Autodesk Inventor part; units mm, degrees
(part 4 of 15)
  line L606 (16.684, 10.808) -> (18.716, 10.808)
  arc A1487 (18.716, 10.7572) -> (18.716, 10.8588) centre (18.716, 10.808) ccw
  arc A1488 (16.684, 10.8588) -> (16.684, 10.7572) centre (16.684, 10.808) ccw
  line L607 (18.716, 10.808) -> (18.716, 9.792)
  arc A1489 (18.6652, 9.792) -> (18.7668, 9.792) centre (18.716, 9.792) ccw
  arc A1490 (18.7668, 10.808) -> (18.6652, 10.808) centre (18.716, 10.808) ccw
  line L608 (18.716, 9.792) -> (16.684, 9.792)
  arc A1491 (16.684, 9.8428) -> (16.684, 9.7412) centre (16.684, 9.792) ccw
  arc A1492 (18.716, 9.7412) -> (18.716, 9.8428) centre (18.716, 9.792) ccw
  line L609 (16.684, 9.792) -> (16.684, 10.808)
  arc A1493 (16.7348, 10.808) -> (16.6332, 10.808) centre (16.684, 10.808) ccw
  arc A1494 (16.6332, 9.792) -> (16.7348, 9.792) centre (16.684, 9.792) ccw
  arc A1495 (39.1348, 45.008) -> (39.0332, 45.008) centre (39.084, 45.008) ccw
  line L610 (22.884, 6.808) -> (24.916, 6.808)
  arc A1496 (24.916, 6.7572) -> (24.916, 6.8588) centre (24.916, 6.808) ccw
  arc A1497 (22.884, 6.8588) -> (22.884, 6.7572) centre (22.884, 6.808) ccw
  line L611 (24.916, 6.808) -> (24.916, 5.792)
  arc A1498 (24.8652, 5.792) -> (24.9668, 5.792) centre (24.916, 5.792) ccw
  arc A1499 (24.9668, 6.808) -> (24.8652, 6.808) centre (24.916, 6.808) ccw
  line L612 (24.916, 5.792) -> (22.884, 5.792)
  arc A1500 (22.884, 5.8428) -> (22.884, 5.7412) centre (22.884, 5.792) ccw
  arc A1501 (24.916, 5.7412) -> (24.916, 5.8428) centre (24.916, 5.792) ccw
  line L613 (22.884, 5.792) -> (22.884, 6.808)
  arc A1502 (22.9348, 6.808) -> (22.8332, 6.808) centre (22.884, 6.808) ccw
  arc A1503 (22.8332, 5.792) -> (22.9348, 5.792) centre (22.884, 5.792) ccw
  arc A1504 (39.0332, 43.992) -> (39.1348, 43.992) centre (39.084, 43.992) ccw
  line L614 (12.684, 13.208) -> (14.716, 13.208)
  arc A1505 (14.716, 13.1572) -> (14.716, 13.2588) centre (14.716, 13.208) ccw
  arc A1506 (12.684, 13.2588) -> (12.684, 13.1572) centre (12.684, 13.208) ccw
  line L615 (14.716, 13.208) -> (14.716, 12.192)
  arc A1507 (14.6652, 12.192) -> (14.7668, 12.192) centre (14.716, 12.192) ccw
  arc A1508 (14.7668, 13.208) -> (14.6652, 13.208) centre (14.716, 13.208) ccw
  line L616 (14.716, 12.192) -> (12.684, 12.192)
  arc A1509 (12.684, 12.2428) -> (12.684, 12.1412) centre (12.684, 12.192) ccw
  arc A1510 (14.716, 12.1412) -> (14.716, 12.2428) centre (14.716, 12.192) ccw
  line L617 (12.684, 12.192) -> (12.684, 13.208)
  arc A1511 (12.7348, 13.208) -> (12.6332, 13.208) centre (12.684, 13.208) ccw
  arc A1512 (12.6332, 12.192) -> (12.7348, 12.192) centre (12.684, 12.192) ccw
  line L618 (39.084, 45.008) -> (41.116, 45.008)
  line L619 (14.684, 13.208) -> (16.716, 13.208)
  arc A1513 (16.716, 13.1572) -> (16.716, 13.2588) centre (16.716, 13.208) ccw
  arc A1514 (14.684, 13.2588) -> (14.684, 13.1572) centre (14.684, 13.208) ccw
  line L620 (16.716, 13.208) -> (16.716, 12.192)
  arc A1515 (16.6652, 12.192) -> (16.7668, 12.192) centre (16.716, 12.192) ccw
  arc A1516 (16.7668, 13.208) -> (16.6652, 13.208) centre (16.716, 13.208) ccw
  line L621 (16.716, 12.192) -> (14.684, 12.192)
  arc A1517 (14.684, 12.2428) -> (14.684, 12.1412) centre (14.684, 12.192) ccw
  arc A1518 (16.716, 12.1412) -> (16.716, 12.2428) centre (16.716, 12.192) ccw
  line L622 (14.684, 12.192) -> (14.684, 13.208)
  arc A1519 (14.7348, 13.208) -> (14.6332, 13.208) centre (14.684, 13.208) ccw
  arc A1520 (14.6332, 12.192) -> (14.7348, 12.192) centre (14.684, 12.192) ccw
  arc A1521 (41.116, 44.9572) -> (41.116, 45.0588) centre (41.116, 45.008) ccw
  line L623 (12.684, 21.208) -> (14.716, 21.208)
  arc A1522 (14.716, 21.1572) -> (14.716, 21.2588) centre (14.716, 21.208) ccw
  arc A1523 (12.684, 21.2588) -> (12.684, 21.1572) centre (12.684, 21.208) ccw
  line L624 (14.716, 21.208) -> (14.716, 20.192)
  arc A1524 (14.6652, 20.192) -> (14.7668, 20.192) centre (14.716, 20.192) ccw
  arc A1525 (14.7668, 21.208) -> (14.6652, 21.208) centre (14.716, 21.208) ccw
  line L625 (14.716, 20.192) -> (12.684, 20.192)
  arc A1526 (12.684, 20.2428) -> (12.684, 20.1412) centre (12.684, 20.192) ccw
  arc A1527 (14.716, 20.1412) -> (14.716, 20.2428) centre (14.716, 20.192) ccw
  line L626 (12.684, 20.192) -> (12.684, 21.208)
  arc A1528 (12.7348, 21.208) -> (12.6332, 21.208) centre (12.684, 21.208) ccw
  arc A1529 (12.6332, 20.192) -> (12.7348, 20.192) centre (12.684, 20.192) ccw
  arc A1530 (39.084, 45.0588) -> (39.084, 44.9572) centre (39.084, 45.008) ccw
  line L627 (12.684, 2.808) -> (14.716, 2.808)
  arc A1531 (14.716, 2.7572) -> (14.716, 2.8588) centre (14.716, 2.808) ccw
  arc A1532 (12.684, 2.8588) -> (12.684, 2.7572) centre (12.684, 2.808) ccw
  line L628 (14.716, 2.808) -> (14.716, 1.792)
  arc A1533 (14.6652, 1.792) -> (14.7668, 1.792) centre (14.716, 1.792) ccw
  arc A1534 (14.7668, 2.808) -> (14.6652, 2.808) centre (14.716, 2.808) ccw
  line L629 (14.716, 1.792) -> (12.684, 1.792)
  arc A1535 (12.684, 1.8428) -> (12.684, 1.7412) centre (12.684, 1.792) ccw
  arc A1536 (14.716, 1.7412) -> (14.716, 1.8428) centre (14.716, 1.792) ccw
  line L630 (12.684, 1.792) -> (12.684, 2.808)
  arc A1537 (12.7348, 2.808) -> (12.6332, 2.808) centre (12.684, 2.808) ccw
  arc A1538 (12.6332, 1.792) -> (12.7348, 1.792) centre (12.684, 1.792) ccw
  line L631 (41.116, 45.008) -> (41.116, 43.992)
  line L632 (14.684, 2.808) -> (16.716, 2.808)
  arc A1539 (16.716, 2.7572) -> (16.716, 2.8588) centre (16.716, 2.808) ccw
  arc A1540 (14.684, 2.8588) -> (14.684, 2.7572) centre (14.684, 2.808) ccw
  line L633 (16.716, 2.808) -> (16.716, 1.792)
  arc A1541 (16.6652, 1.792) -> (16.7668, 1.792) centre (16.716, 1.792) ccw
  arc A1542 (16.7668, 2.808) -> (16.6652, 2.808) centre (16.716, 2.808) ccw
  line L634 (16.716, 1.792) -> (14.684, 1.792)
  arc A1543 (14.684, 1.8428) -> (14.684, 1.7412) centre (14.684, 1.792) ccw
  arc A1544 (16.716, 1.7412) -> (16.716, 1.8428) centre (16.716, 1.792) ccw
  line L635 (14.684, 1.792) -> (14.684, 2.808)
  arc A1545 (14.7348, 2.808) -> (14.6332, 2.808) centre (14.684, 2.808) ccw
  arc A1546 (14.6332, 1.792) -> (14.7348, 1.792) centre (14.684, 1.792) ccw
  arc A1547 (41.0652, 43.992) -> (41.1668, 43.992) centre (41.116, 43.992) ccw
  line L636 (12.684, 10.808) -> (14.716, 10.808)
  arc A1548 (14.716, 10.7572) -> (14.716, 10.8588) centre (14.716, 10.808) ccw
  arc A1549 (12.684, 10.8588) -> (12.684, 10.7572) centre (12.684, 10.808) ccw
  line L637 (14.716, 10.808) -> (14.716, 9.792)
  arc A1550 (14.6652, 9.792) -> (14.7668, 9.792) centre (14.716, 9.792) ccw
  arc A1551 (14.7668, 10.808) -> (14.6652, 10.808) centre (14.716, 10.808) ccw
  line L638 (14.716, 9.792) -> (12.684, 9.792)
  arc A1552 (12.684, 9.8428) -> (12.684, 9.7412) centre (12.684, 9.792) ccw
  arc A1553 (14.716, 9.7412) -> (14.716, 9.8428) centre (14.716, 9.792) ccw
  line L639 (12.684, 9.792) -> (12.684, 10.808)
  arc A1554 (12.7348, 10.808) -> (12.6332, 10.808) centre (12.684, 10.808) ccw
  arc A1555 (12.6332, 9.792) -> (12.7348, 9.792) centre (12.684, 9.792) ccw
  arc A1556 (41.1668, 45.008) -> (41.0652, 45.008) centre (41.116, 45.008) ccw
  line L640 (14.684, 21.208) -> (16.716, 21.208)
  arc A1557 (16.716, 21.1572) -> (16.716, 21.2588) centre (16.716, 21.208) ccw
  arc A1558 (14.684, 21.2588) -> (14.684, 21.1572) centre (14.684, 21.208) ccw
  line L641 (16.716, 21.208) -> (16.716, 20.192)
  arc A1559 (16.6652, 20.192) -> (16.7668, 20.192) centre (16.716, 20.192) ccw
  arc A1560 (16.7668, 21.208) -> (16.6652, 21.208) centre (16.716, 21.208) ccw
  line L642 (16.716, 20.192) -> (14.684, 20.192)
  arc A1561 (14.684, 20.2428) -> (14.684, 20.1412) centre (14.684, 20.192) ccw
  arc A1562 (16.716, 20.1412) -> (16.716, 20.2428) centre (16.716, 20.192) ccw
  line L643 (14.684, 20.192) -> (14.684, 21.208)
  arc A1563 (14.7348, 21.208) -> (14.6332, 21.208) centre (14.684, 21.208) ccw
  arc A1564 (14.6332, 20.192) -> (14.7348, 20.192) centre (14.684, 20.192) ccw
  line L644 (41.116, 42.992) -> (39.084, 42.992)
  line L645 (16.716, 16.192) -> (14.684, 16.192)
  arc A1565 (14.684, 16.2428) -> (14.684, 16.1412) centre (14.684, 16.192) ccw
  arc A1566 (16.716, 16.1412) -> (16.716, 16.2428) centre (16.716, 16.192) ccw
  line L646 (14.684, 16.192) -> (14.684, 17.208)
  arc A1567 (14.7348, 17.208) -> (14.6332, 17.208) centre (14.684, 17.208) ccw
  arc A1568 (14.6332, 16.192) -> (14.7348, 16.192) centre (14.684, 16.192) ccw
  line L647 (14.684, 17.208) -> (16.716, 17.208)
  arc A1569 (16.716, 17.1572) -> (16.716, 17.2588) centre (16.716, 17.208) ccw
  arc A1570 (14.684, 17.2588) -> (14.684, 17.1572) centre (14.684, 17.208) ccw
  line L648 (16.716, 17.208) -> (16.716, 16.192)
  arc A1571 (16.6652, 16.192) -> (16.7668, 16.192) centre (16.716, 16.192) ccw
  arc A1572 (16.7668, 17.208) -> (16.6652, 17.208) centre (16.716, 17.208) ccw
  arc A1573 (39.084, 43.0428) -> (39.084, 42.9412) centre (39.084, 42.992) ccw
  line L649 (22.884, 13.208) -> (24.916, 13.208)
  arc A1574 (24.916, 13.1572) -> (24.916, 13.2588) centre (24.916, 13.208) ccw
  arc A1575 (22.884, 13.2588) -> (22.884, 13.1572) centre (22.884, 13.208) ccw
  line L650 (24.916, 13.208) -> (24.916, 12.192)
  arc A1576 (24.8652, 12.192) -> (24.9668, 12.192) centre (24.916, 12.192) ccw
  arc A1577 (24.9668, 13.208) -> (24.8652, 13.208) centre (24.916, 13.208) ccw
  line L651 (24.916, 12.192) -> (22.884, 12.192)
  arc A1578 (22.884, 12.2428) -> (22.884, 12.1412) centre (22.884, 12.192) ccw
  arc A1579 (24.916, 12.1412) -> (24.916, 12.2428) centre (24.916, 12.192) ccw
  line L652 (22.884, 12.192) -> (22.884, 13.208)
  arc A1580 (22.9348, 13.208) -> (22.8332, 13.208) centre (22.884, 13.208) ccw
  arc A1581 (22.8332, 12.192) -> (22.9348, 12.192) centre (22.884, 12.192) ccw
  arc A1582 (41.116, 42.9412) -> (41.116, 43.0428) centre (41.116, 42.992) ccw
  line L653 (14.684, 10.808) -> (16.716, 10.808)
  arc A1583 (16.716, 10.7572) -> (16.716, 10.8588) centre (16.716, 10.808) ccw
  arc A1584 (14.684, 10.8588) -> (14.684, 10.7572) centre (14.684, 10.808) ccw
  line L654 (16.716, 10.808) -> (16.716, 9.792)
  arc A1585 (16.6652, 9.792) -> (16.7668, 9.792) centre (16.716, 9.792) ccw
  arc A1586 (16.7668, 10.808) -> (16.6652, 10.808) centre (16.716, 10.808) ccw
  line L655 (16.716, 9.792) -> (14.684, 9.792)
  arc A1587 (14.684, 9.8428) -> (14.684, 9.7412) centre (14.684, 9.792) ccw
  arc A1588 (16.716, 9.7412) -> (16.716, 9.8428) centre (16.716, 9.792) ccw
  line L656 (14.684, 9.792) -> (14.684, 10.808)
  arc A1589 (14.7348, 10.808) -> (14.6332, 10.808) centre (14.684, 10.808) ccw
  arc A1590 (14.6332, 9.792) -> (14.7348, 9.792) centre (14.684, 9.792) ccw
  line L657 (39.084, 42.992) -> (39.084, 44.008)
  line L658 (16.716, 5.692) -> (14.684, 5.692)
  arc A1591 (14.684, 5.7428) -> (14.684, 5.6412) centre (14.684, 5.692) ccw
  arc A1592 (16.716, 5.6412) -> (16.716, 5.7428) centre (16.716, 5.692) ccw
  line L659 (14.684, 5.692) -> (14.684, 6.708)
  arc A1593 (14.7348, 6.708) -> (14.6332, 6.708) centre (14.684, 6.708) ccw
  arc A1594 (14.6332, 5.692) -> (14.7348, 5.692) centre (14.684, 5.692) ccw
  line L660 (14.684, 6.708) -> (16.716, 6.708)
  arc A1595 (16.716, 6.6572) -> (16.716, 6.7588) centre (16.716, 6.708) ccw
  arc A1596 (14.684, 6.7588) -> (14.684, 6.6572) centre (14.684, 6.708) ccw
  line L661 (16.716, 6.708) -> (16.716, 5.692)
  arc A1597 (16.6652, 5.692) -> (16.7668, 5.692) centre (16.716, 5.692) ccw
  arc A1598 (16.7668, 6.708) -> (16.6652, 6.708) centre (16.716, 6.708) ccw
  arc A1599 (39.1348, 44.008) -> (39.0332, 44.008) centre (39.084, 44.008) ccw
  line L662 (22.884, 2.808) -> (24.916, 2.808)
  arc A1600 (24.916, 2.7572) -> (24.916, 2.8588) centre (24.916, 2.808) ccw
  arc A1601 (22.884, 2.8588) -> (22.884, 2.7572) centre (22.884, 2.808) ccw
  line L663 (24.916, 2.808) -> (24.916, 1.792)
  arc A1602 (24.8652, 1.792) -> (24.9668, 1.792) centre (24.916, 1.792) ccw
  arc A1603 (24.9668, 2.808) -> (24.8652, 2.808) centre (24.916, 2.808) ccw
  line L664 (24.916, 1.792) -> (22.884, 1.792)
  arc A1604 (22.884, 1.8428) -> (22.884, 1.7412) centre (22.884, 1.792) ccw
  arc A1605 (24.916, 1.7412) -> (24.916, 1.8428) centre (24.916, 1.792) ccw
  line L665 (22.884, 1.792) -> (22.884, 2.808)
  arc A1606 (22.9348, 2.808) -> (22.8332, 2.808) centre (22.884, 2.808) ccw
  arc A1607 (22.8332, 1.792) -> (22.9348, 1.792) centre (22.884, 1.792) ccw
  arc A1608 (39.0332, 42.992) -> (39.1348, 42.992) centre (39.084, 42.992) ccw
  line L666 (20.916, 12.192) -> (18.884, 12.192)
  arc A1609 (18.884, 12.2428) -> (18.884, 12.1412) centre (18.884, 12.192) ccw
  arc A1610 (20.916, 12.1412) -> (20.916, 12.2428) centre (20.916, 12.192) ccw
  line L667 (18.884, 12.192) -> (18.884, 13.208)
  arc A1611 (18.9348, 13.208) -> (18.8332, 13.208) centre (18.884, 13.208) ccw
  arc A1612 (18.8332, 12.192) -> (18.9348, 12.192) centre (18.884, 12.192) ccw
  line L668 (18.884, 13.208) -> (20.916, 13.208)
  arc A1613 (20.916, 13.1572) -> (20.916, 13.2588) centre (20.916, 13.208) ccw
  arc A1614 (18.884, 13.2588) -> (18.884, 13.1572) centre (18.884, 13.208) ccw
  line L669 (20.916, 13.208) -> (20.916, 12.192)
  arc A1615 (20.8652, 12.192) -> (20.9668, 12.192) centre (20.916, 12.192) ccw
  arc A1616 (20.9668, 13.208) -> (20.8652, 13.208) centre (20.916, 13.208) ccw
  line L670 (39.084, 44.008) -> (41.116, 44.008)
  line L671 (12.684, 17.208) -> (14.716, 17.208)
  arc A1617 (14.716, 17.1572) -> (14.716, 17.2588) centre (14.716, 17.208) ccw
  arc A1618 (12.684, 17.2588) -> (12.684, 17.1572) centre (12.684, 17.208) ccw
  line L672 (14.716, 17.208) -> (14.716, 16.192)
  arc A1619 (14.6652, 16.192) -> (14.7668, 16.192) centre (14.716, 16.192) ccw
  arc A1620 (14.7668, 17.208) -> (14.6652, 17.208) centre (14.716, 17.208) ccw
  line L673 (14.716, 16.192) -> (12.684, 16.192)
  arc A1621 (12.684, 16.2428) -> (12.684, 16.1412) centre (12.684, 16.192) ccw
  arc A1622 (14.716, 16.1412) -> (14.716, 16.2428) centre (14.716, 16.192) ccw
  line L674 (12.684, 16.192) -> (12.684, 17.208)
  arc A1623 (12.7348, 17.208) -> (12.6332, 17.208) centre (12.684, 17.208) ccw
  arc A1624 (12.6332, 16.192) -> (12.7348, 16.192) centre (12.684, 16.192) ccw
  arc A1625 (41.116, 43.9572) -> (41.116, 44.0588) centre (41.116, 44.008) ccw
  line L675 (20.884, 21.208) -> (22.916, 21.208)
  arc A1626 (22.916, 21.1572) -> (22.916, 21.2588) centre (22.916, 21.208) ccw
  arc A1627 (20.884, 21.2588) -> (20.884, 21.1572) centre (20.884, 21.208) ccw
  line L676 (22.916, 21.208) -> (22.916, 20.192)
  arc A1628 (22.8652, 20.192) -> (22.9668, 20.192) centre (22.916, 20.192) ccw
  arc A1629 (22.9668, 21.208) -> (22.8652, 21.208) centre (22.916, 21.208) ccw
  line L677 (22.916, 20.192) -> (20.884, 20.192)
  arc A1630 (20.884, 20.2428) -> (20.884, 20.1412) centre (20.884, 20.192) ccw
  arc A1631 (22.916, 20.1412) -> (22.916, 20.2428) centre (22.916, 20.192) ccw
  line L678 (20.884, 20.192) -> (20.884, 21.208)
  arc A1632 (20.9348, 21.208) -> (20.8332, 21.208) centre (20.884, 21.208) ccw
  arc A1633 (20.8332, 20.192) -> (20.9348, 20.192) centre (20.884, 20.192) ccw
  arc A1634 (39.084, 44.0588) -> (39.084, 43.9572) centre (39.084, 44.008) ccw
  line L679 (18.884, 2.808) -> (20.916, 2.808)
  arc A1635 (20.916, 2.7572) -> (20.916, 2.8588) centre (20.916, 2.808) ccw
  arc A1636 (18.884, 2.8588) -> (18.884, 2.7572) centre (18.884, 2.808) ccw
  line L680 (20.916, 2.808) -> (20.916, 1.792)
  arc A1637 (20.8652, 1.792) -> (20.9668, 1.792) centre (20.916, 1.792) ccw
  arc A1638 (20.9668, 2.808) -> (20.8652, 2.808) centre (20.916, 2.808) ccw
  line L681 (20.916, 1.792) -> (18.884, 1.792)
  arc A1639 (18.884, 1.8428) -> (18.884, 1.7412) centre (18.884, 1.792) ccw
  arc A1640 (20.916, 1.7412) -> (20.916, 1.8428) centre (20.916, 1.792) ccw
  line L682 (18.884, 1.792) -> (18.884, 2.808)
  arc A1641 (18.9348, 2.808) -> (18.8332, 2.808) centre (18.884, 2.808) ccw
  arc A1642 (18.8332, 1.792) -> (18.9348, 1.792) centre (18.884, 1.792) ccw
  line L683 (41.116, 44.008) -> (41.116, 42.992)
  line L684 (12.684, 6.708) -> (14.716, 6.708)
  arc A1643 (14.716, 6.6572) -> (14.716, 6.7588) centre (14.716, 6.708) ccw
  arc A1644 (12.684, 6.7588) -> (12.684, 6.6572) centre (12.684, 6.708) ccw
  line L685 (14.716, 6.708) -> (14.716, 5.692)
  arc A1645 (14.6652, 5.692) -> (14.7668, 5.692) centre (14.716, 5.692) ccw
  arc A1646 (14.7668, 6.708) -> (14.6652, 6.708) centre (14.716, 6.708) ccw
  line L686 (14.716, 5.692) -> (12.684, 5.692)
  arc A1647 (12.684, 5.7428) -> (12.684, 5.6412) centre (12.684, 5.692) ccw
  arc A1648 (14.716, 5.6412) -> (14.716, 5.7428) centre (14.716, 5.692) ccw
  line L687 (12.684, 5.692) -> (12.684, 6.708)
  arc A1649 (12.7348, 6.708) -> (12.6332, 6.708) centre (12.684, 6.708) ccw
  arc A1650 (12.6332, 5.692) -> (12.7348, 5.692) centre (12.684, 5.692) ccw
  arc A1651 (41.0652, 42.992) -> (41.1668, 42.992) centre (41.116, 42.992) ccw
  line L688 (20.884, 10.808) -> (22.916, 10.808)
  arc A1652 (22.916, 10.7572) -> (22.916, 10.8588) centre (22.916, 10.808) ccw
  arc A1653 (20.884, 10.8588) -> (20.884, 10.7572) centre (20.884, 10.808) ccw
  line L689 (22.916, 10.808) -> (22.916, 9.792)
  arc A1654 (22.8652, 9.792) -> (22.9668, 9.792) centre (22.916, 9.792) ccw
  arc A1655 (22.9668, 10.808) -> (22.8652, 10.808) centre (22.916, 10.808) ccw
  line L690 (22.916, 9.792) -> (20.884, 9.792)
  arc A1656 (20.884, 9.8428) -> (20.884, 9.7412) centre (20.884, 9.792) ccw
  arc A1657 (22.916, 9.7412) -> (22.916, 9.8428) centre (22.916, 9.792) ccw
  line L691 (20.884, 9.792) -> (20.884, 10.808)
  arc A1658 (20.9348, 10.808) -> (20.8332, 10.808) centre (20.884, 10.808) ccw
  arc A1659 (20.8332, 9.792) -> (20.9348, 9.792) centre (20.884, 9.792) ccw
  arc A1660 (41.1668, 44.008) -> (41.0652, 44.008) centre (41.116, 44.008) ccw
  line L692 (22.884, 21.208) -> (24.916, 21.208)
  arc A1661 (24.916, 21.1572) -> (24.916, 21.2588) centre (24.916, 21.208) ccw
  arc A1662 (22.884, 21.2588) -> (22.884, 21.1572) centre (22.884, 21.208) ccw
  line L693 (24.916, 21.208) -> (24.916, 20.192)
  arc A1663 (24.8652, 20.192) -> (24.9668, 20.192) centre (24.916, 20.192) ccw
  arc A1664 (24.9668, 21.208) -> (24.8652, 21.208) centre (24.916, 21.208) ccw
  line L694 (24.916, 20.192) -> (22.884, 20.192)
  arc A1665 (22.884, 20.2428) -> (22.884, 20.1412) centre (22.884, 20.192) ccw
  arc A1666 (24.916, 20.1412) -> (24.916, 20.2428) centre (24.916, 20.192) ccw
  line L695 (22.884, 20.192) -> (22.884, 21.208)
  arc A1667 (22.9348, 21.208) -> (22.8332, 21.208) centre (22.884, 21.208) ccw
  arc A1668 (22.8332, 20.192) -> (22.9348, 20.192) centre (22.884, 20.192) ccw
  line L696 (68.816, 35.092) -> (66.784, 35.092)
  line L697 (18.684, 17.208) -> (20.716, 17.208)
  arc A1669 (20.716, 17.1572) -> (20.716, 17.2588) centre (20.716, 17.208) ccw
  arc A1670 (18.684, 17.2588) -> (18.684, 17.1572) centre (18.684, 17.208) ccw
  line L698 (20.716, 17.208) -> (20.716, 16.192)
  arc A1671 (20.6652, 16.192) -> (20.7668, 16.192) centre (20.716, 16.192) ccw
  arc A1672 (20.7668, 17.208) -> (20.6652, 17.208) centre (20.716, 17.208) ccw
  line L699 (20.716, 16.192) -> (18.684, 16.192)
  arc A1673 (18.684, 16.2428) -> (18.684, 16.1412) centre (18.684, 16.192) ccw
  arc A1674 (20.716, 16.1412) -> (20.716, 16.2428) centre (20.716, 16.192) ccw
  line L700 (18.684, 16.192) -> (18.684, 17.208)
  arc A1675 (18.7348, 17.208) -> (18.6332, 17.208) centre (18.684, 17.208) ccw
  arc A1676 (18.6332, 16.192) -> (18.7348, 16.192) centre (18.684, 16.192) ccw
  arc A1677 (66.784, 35.1428) -> (66.784, 35.0412) centre (66.784, 35.092) ccw
  line L701 (22.884, 10.808) -> (24.916, 10.808)
  arc A1678 (24.916, 10.7572) -> (24.916, 10.8588) centre (24.916, 10.808) ccw
  arc A1679 (22.884, 10.8588) -> (22.884, 10.7572) centre (22.884, 10.808) ccw
  line L702 (24.916, 10.808) -> (24.916, 9.792)
  arc A1680 (24.8652, 9.792) -> (24.9668, 9.792) centre (24.916, 9.792) ccw
  arc A1681 (24.9668, 10.808) -> (24.8652, 10.808) centre (24.916, 10.808) ccw
  line L703 (24.916, 9.792) -> (22.884, 9.792)
  arc A1682 (22.884, 9.8428) -> (22.884, 9.7412) centre (22.884, 9.792) ccw
  arc A1683 (24.916, 9.7412) -> (24.916, 9.8428) centre (24.916, 9.792) ccw
  line L704 (22.884, 9.792) -> (22.884, 10.808)
  arc A1684 (22.9348, 10.808) -> (22.8332, 10.808) centre (22.884, 10.808) ccw
  arc A1685 (22.8332, 9.792) -> (22.9348, 9.792) centre (22.884, 9.792) ccw
  arc A1686 (68.816, 35.0412) -> (68.816, 35.1428) centre (68.816, 35.092) ccw
  line L705 (18.684, 6.708) -> (20.716, 6.708)
  arc A1687 (20.716, 6.6572) -> (20.716, 6.7588) centre (20.716, 6.708) ccw
  arc A1688 (18.684, 6.7588) -> (18.684, 6.6572) centre (18.684, 6.708) ccw
  line L706 (20.716, 6.708) -> (20.716, 5.692)
  arc A1689 (20.6652, 5.692) -> (20.7668, 5.692) centre (20.716, 5.692) ccw
  arc A1690 (20.7668, 6.708) -> (20.6652, 6.708) centre (20.716, 6.708) ccw
  line L707 (20.716, 5.692) -> (18.684, 5.692)
  arc A1691 (18.684, 5.7428) -> (18.684, 5.6412) centre (18.684, 5.692) ccw
  arc A1692 (20.716, 5.6412) -> (20.716, 5.7428) centre (20.716, 5.692) ccw
  line L708 (18.684, 5.692) -> (18.684, 6.708)
  arc A1693 (18.7348, 6.708) -> (18.6332, 6.708) centre (18.684, 6.708) ccw
  arc A1694 (18.6332, 5.692) -> (18.7348, 5.692) centre (18.684, 5.692) ccw
  line L709 (66.784, 35.092) -> (66.784, 36.108)
  line L710 (20.916, -0.608) -> (18.884, -0.608)
  arc A1695 (18.884, -0.5572) -> (18.884, -0.6588) centre (18.884, -0.608) ccw
  arc A1696 (20.916, -0.6588) -> (20.916, -0.5572) centre (20.916, -0.608) ccw
  line L711 (18.884, -0.608) -> (18.884, 0.408)
  arc A1697 (18.9348, 0.408) -> (18.8332, 0.408) centre (18.884, 0.408) ccw
  arc A1698 (18.8332, -0.608) -> (18.9348, -0.608) centre (18.884, -0.608) ccw
  line L712 (18.884, 0.408) -> (20.916, 0.408)
  arc A1699 (20.916, 0.3572) -> (20.916, 0.4588) centre (20.916, 0.408) ccw
  arc A1700 (18.884, 0.4588) -> (18.884, 0.3572) centre (18.884, 0.408) ccw
  line L713 (20.916, 0.408) -> (20.916, -0.608)
  arc A1701 (20.8652, -0.608) -> (20.9668, -0.608) centre (20.916, -0.608) ccw
  arc A1702 (20.9668, 0.408) -> (20.8652, 0.408) centre (20.916, 0.408) ccw
  arc A1703 (66.8348, 36.108) -> (66.7332, 36.108) centre (66.784, 36.108) ccw
  line L714 (16.684, 0.408) -> (18.716, 0.408)
  arc A1704 (18.716, 0.3572) -> (18.716, 0.4588) centre (18.716, 0.408) ccw
  arc A1705 (16.684, 0.4588) -> (16.684, 0.3572) centre (16.684, 0.408) ccw
  line L715 (18.716, 0.408) -> (18.716, -0.608)
  arc A1706 (18.6652, -0.608) -> (18.7668, -0.608) centre (18.716, -0.608) ccw
  arc A1707 (18.7668, 0.408) -> (18.6652, 0.408) centre (18.716, 0.408) ccw
  line L716 (18.716, -0.608) -> (16.684, -0.608)
  arc A1708 (16.684, -0.5572) -> (16.684, -0.6588) centre (16.684, -0.608) ccw
  arc A1709 (18.716, -0.6588) -> (18.716, -0.5572) centre (18.716, -0.608) ccw
  line L717 (16.684, -0.608) -> (16.684, 0.408)
  arc A1710 (16.7348, 0.408) -> (16.6332, 0.408) centre (16.684, 0.408) ccw
  arc A1711 (16.6332, -0.608) -> (16.7348, -0.608) centre (16.684, -0.608) ccw
  arc A1712 (66.7332, 35.092) -> (66.8348, 35.092) centre (66.784, 35.092) ccw
  line L718 (22.884, -3.592) -> (24.916, -3.592)
  arc A1713 (24.916, -3.6428) -> (24.916, -3.5412) centre (24.916, -3.592) ccw
  arc A1714 (22.884, -3.5412) -> (22.884, -3.6428) centre (22.884, -3.592) ccw
  line L719 (24.916, -3.592) -> (24.916, -4.608)
  arc A1715 (24.8652, -4.608) -> (24.9668, -4.608) centre (24.916, -4.608) ccw
  arc A1716 (24.9668, -3.592) -> (24.8652, -3.592) centre (24.916, -3.592) ccw
  line L720 (24.916, -4.608) -> (22.884, -4.608)
  arc A1717 (22.884, -4.5572) -> (22.884, -4.6588) centre (22.884, -4.608) ccw
  arc A1718 (24.916, -4.6588) -> (24.916, -4.5572) centre (24.916, -4.608) ccw
  line L721 (22.884, -4.608) -> (22.884, -3.592)
  arc A1719 (22.9348, -3.592) -> (22.8332, -3.592) centre (22.884, -3.592) ccw
  arc A1720 (22.8332, -4.608) -> (22.9348, -4.608) centre (22.884, -4.608) ccw
  line L722 (66.784, 36.108) -> (68.816, 36.108)
  line L723 (20.916, -11.008) -> (18.884, -11.008)
  arc A1721 (18.884, -10.9572) -> (18.884, -11.0588) centre (18.884, -11.008) ccw
  arc A1722 (20.916, -11.0588) -> (20.916, -10.9572) centre (20.916, -11.008) ccw
  line L724 (18.884, -11.008) -> (18.884, -9.992)
  arc A1723 (18.9348, -9.992) -> (18.8332, -9.992) centre (18.884, -9.992) ccw
  arc A1724 (18.8332, -11.008) -> (18.9348, -11.008) centre (18.884, -11.008) ccw
  line L725 (18.884, -9.992) -> (20.916, -9.992)
  arc A1725 (20.916, -10.0428) -> (20.916, -9.9412) centre (20.916, -9.992) ccw
  arc A1726 (18.884, -9.9412) -> (18.884, -10.0428) centre (18.884, -9.992) ccw
  line L726 (20.916, -9.992) -> (20.916, -11.008)
  arc A1727 (20.8652, -11.008) -> (20.9668, -11.008) centre (20.916, -11.008) ccw
  arc A1728 (20.9668, -9.992) -> (20.8652, -9.992) centre (20.916, -9.992) ccw
  arc A1729 (68.816, 36.0572) -> (68.816, 36.1588) centre (68.816, 36.108) ccw
  line L727 (16.684, -9.992) -> (18.716, -9.992)
  arc A1730 (18.716, -10.0428) -> (18.716, -9.9412) centre (18.716, -9.992) ccw
  arc A1731 (16.684, -9.9412) -> (16.684, -10.0428) centre (16.684, -9.992) ccw
  line L728 (18.716, -9.992) -> (18.716, -11.008)
  arc A1732 (18.6652, -11.008) -> (18.7668, -11.008) centre (18.716, -11.008) ccw
  arc A1733 (18.7668, -9.992) -> (18.6652, -9.992) centre (18.716, -9.992) ccw
  line L729 (18.716, -11.008) -> (16.684, -11.008)
  arc A1734 (16.684, -10.9572) -> (16.684, -11.0588) centre (16.684, -11.008) ccw
  arc A1735 (18.716, -11.0588) -> (18.716, -10.9572) centre (18.716, -11.008) ccw
  line L730 (16.684, -11.008) -> (16.684, -9.992)
  arc A1736 (16.7348, -9.992) -> (16.6332, -9.992) centre (16.684, -9.992) ccw
  arc A1737 (16.6332, -11.008) -> (16.7348, -11.008) centre (16.684, -11.008) ccw
  arc A1738 (66.784, 36.1588) -> (66.784, 36.0572) centre (66.784, 36.108) ccw
  line L731 (22.884, -13.992) -> (24.916, -13.992)
  arc A1739 (24.916, -14.0428) -> (24.916, -13.9412) centre (24.916, -13.992) ccw
  arc A1740 (22.884, -13.9412) -> (22.884, -14.0428) centre (22.884, -13.992) ccw
  line L732 (24.916, -13.992) -> (24.916, -15.008)
  arc A1741 (24.8652, -15.008) -> (24.9668, -15.008) centre (24.916, -15.008) ccw
  arc A1742 (24.9668, -13.992) -> (24.8652, -13.992) centre (24.916, -13.992) ccw
  line L733 (24.916, -15.008) -> (22.884, -15.008)
  arc A1743 (22.884, -14.9572) -> (22.884, -15.0588) centre (22.884, -15.008) ccw
  arc A1744 (24.916, -15.0588) -> (24.916, -14.9572) centre (24.916, -15.008) ccw
  line L734 (22.884, -15.008) -> (22.884, -13.992)
  arc A1745 (22.9348, -13.992) -> (22.8332, -13.992) centre (22.884, -13.992) ccw
  arc A1746 (22.8332, -15.008) -> (22.9348, -15.008) centre (22.884, -15.008) ccw
  line L735 (68.816, 36.108) -> (68.816, 35.092)
  line L736 (12.684, -7.592) -> (14.716, -7.592)
  arc A1747 (14.716, -7.6428) -> (14.716, -7.5412) centre (14.716, -7.592) ccw
  arc A1748 (12.684, -7.5412) -> (12.684, -7.6428) centre (12.684, -7.592) ccw
  line L737 (14.716, -7.592) -> (14.716, -8.608)
  arc A1749 (14.6652, -8.608) -> (14.7668, -8.608) centre (14.716, -8.608) ccw
  arc A1750 (14.7668, -7.592) -> (14.6652, -7.592) centre (14.716, -7.592) ccw
  line L738 (14.716, -8.608) -> (12.684, -8.608)
  arc A1751 (12.684, -8.5572) -> (12.684, -8.6588) centre (12.684, -8.608) ccw
  arc A1752 (14.716, -8.6588) -> (14.716, -8.5572) centre (14.716, -8.608) ccw
  line L739 (12.684, -8.608) -> (12.684, -7.592)
  arc A1753 (12.7348, -7.592) -> (12.6332, -7.592) centre (12.684, -7.592) ccw
  arc A1754 (12.6332, -8.608) -> (12.7348, -8.608) centre (12.684, -8.608) ccw
  arc A1755 (68.7652, 35.092) -> (68.8668, 35.092) centre (68.816, 35.092) ccw
  line L740 (14.684, -7.592) -> (16.716, -7.592)
  arc A1756 (16.716, -7.6428) -> (16.716, -7.5412) centre (16.716, -7.592) ccw
  arc A1757 (14.684, -7.5412) -> (14.684, -7.6428) centre (14.684, -7.592) ccw
  line L741 (16.716, -7.592) -> (16.716, -8.608)
  arc A1758 (16.6652, -8.608) -> (16.7668, -8.608) centre (16.716, -8.608) ccw
  arc A1759 (16.7668, -7.592) -> (16.6652, -7.592) centre (16.716, -7.592) ccw
  line L742 (16.716, -8.608) -> (14.684, -8.608)
  arc A1760 (14.684, -8.5572) -> (14.684, -8.6588) centre (14.684, -8.608) ccw
  arc A1761 (16.716, -8.6588) -> (16.716, -8.5572) centre (16.716, -8.608) ccw
  line L743 (14.684, -8.608) -> (14.684, -7.592)
  arc A1762 (14.7348, -7.592) -> (14.6332, -7.592) centre (14.684, -7.592) ccw
  arc A1763 (14.6332, -8.608) -> (14.7348, -8.608) centre (14.684, -8.608) ccw
  arc A1764 (68.8668, 36.108) -> (68.7652, 36.108) centre (68.816, 36.108) ccw
  line L744 (12.684, 0.408) -> (14.716, 0.408)
  arc A1765 (14.716, 0.3572) -> (14.716, 0.4588) centre (14.716, 0.408) ccw
  arc A1766 (12.684, 0.4588) -> (12.684, 0.3572) centre (12.684, 0.408) ccw
  line L745 (14.716, 0.408) -> (14.716, -0.608)
  arc A1767 (14.6652, -0.608) -> (14.7668, -0.608) centre (14.716, -0.608) ccw
  arc A1768 (14.7668, 0.408) -> (14.6652, 0.408) centre (14.716, 0.408) ccw
  line L746 (14.716, -0.608) -> (12.684, -0.608)
  arc A1769 (12.684, -0.5572) -> (12.684, -0.6588) centre (12.684, -0.608) ccw
  arc A1770 (14.716, -0.6588) -> (14.716, -0.5572) centre (14.716, -0.608) ccw
  line L747 (12.684, -0.608) -> (12.684, 0.408)
  arc A1771 (12.7348, 0.408) -> (12.6332, 0.408) centre (12.684, 0.408) ccw
  arc A1772 (12.6332, -0.608) -> (12.7348, -0.608) centre (12.684, -0.608) ccw
  line L748 (68.816, 39.092) -> (66.784, 39.092)
  line L749 (12.684, -17.992) -> (14.716, -17.992)
  arc A1773 (14.716, -18.0428) -> (14.716, -17.9412) centre (14.716, -17.992) ccw
  arc A1774 (12.684, -17.9412) -> (12.684, -18.0428) centre (12.684, -17.992) ccw
  line L750 (14.716, -17.992) -> (14.716, -19.008)
  arc A1775 (14.6652, -19.008) -> (14.7668, -19.008) centre (14.716, -19.008) ccw
  arc A1776 (14.7668, -17.992) -> (14.6652, -17.992) centre (14.716, -17.992) ccw
  line L751 (14.716, -19.008) -> (12.684, -19.008)
  arc A1777 (12.684, -18.9572) -> (12.684, -19.0588) centre (12.684, -19.008) ccw
  arc A1778 (14.716, -19.0588) -> (14.716, -18.9572) centre (14.716, -19.008) ccw
  line L752 (12.684, -19.008) -> (12.684, -17.992)
  arc A1779 (12.7348, -17.992) -> (12.6332, -17.992) centre (12.684, -17.992) ccw
  arc A1780 (12.6332, -19.008) -> (12.7348, -19.008) centre (12.684, -19.008) ccw
  arc A1781 (66.784, 39.1428) -> (66.784, 39.0412) centre (66.784, 39.092) ccw
  line L753 (14.684, -17.992) -> (16.716, -17.992)
  arc A1782 (16.716, -18.0428) -> (16.716, -17.9412) centre (16.716, -17.992) ccw
  arc A1783 (14.684, -17.9412) -> (14.684, -18.0428) centre (14.684, -17.992) ccw
  line L754 (16.716, -17.992) -> (16.716, -19.008)
  arc A1784 (16.6652, -19.008) -> (16.7668, -19.008) centre (16.716, -19.008) ccw
  arc A1785 (16.7668, -17.992) -> (16.6652, -17.992) centre (16.716, -17.992) ccw
  line L755 (16.716, -19.008) -> (14.684, -19.008)
  arc A1786 (14.684, -18.9572) -> (14.684, -19.0588) centre (14.684, -19.008) ccw
  arc A1787 (16.716, -19.0588) -> (16.716, -18.9572) centre (16.716, -19.008) ccw
  line L756 (14.684, -19.008) -> (14.684, -17.992)
  arc A1788 (14.7348, -17.992) -> (14.6332, -17.992) centre (14.684, -17.992) ccw
  arc A1789 (14.6332, -19.008) -> (14.7348, -19.008) centre (14.684, -19.008) ccw
  arc A1790 (68.816, 39.0412) -> (68.816, 39.1428) centre (68.816, 39.092) ccw
  line L757 (12.684, -9.992) -> (14.716, -9.992)
  arc A1791 (14.716, -10.0428) -> (14.716, -9.9412) centre (14.716, -9.992) ccw
  arc A1792 (12.684, -9.9412) -> (12.684, -10.0428) centre (12.684, -9.992) ccw
  line L758 (14.716, -9.992) -> (14.716, -11.008)
  arc A1793 (14.6652, -11.008) -> (14.7668, -11.008) centre (14.716, -11.008) ccw
  arc A1794 (14.7668, -9.992) -> (14.6652, -9.992) centre (14.716, -9.992) ccw
  line L759 (14.716, -11.008) -> (12.684, -11.008)
  arc A1795 (12.684, -10.9572) -> (12.684, -11.0588) centre (12.684, -11.008) ccw
  arc A1796 (14.716, -11.0588) -> (14.716, -10.9572) centre (14.716, -11.008) ccw
  line L760 (12.684, -11.008) -> (12.684, -9.992)
  arc A1797 (12.7348, -9.992) -> (12.6332, -9.992) centre (12.684, -9.992) ccw
  arc A1798 (12.6332, -11.008) -> (12.7348, -11.008) centre (12.684, -11.008) ccw
  line L761 (66.784, 39.092) -> (66.784, 40.108)
  line L762 (14.684, 0.408) -> (16.716, 0.408)
  arc A1799 (16.716, 0.3572) -> (16.716, 0.4588) centre (16.716, 0.408) ccw
  arc A1800 (14.684, 0.4588) -> (14.684, 0.3572) centre (14.684, 0.408) ccw
  line L763 (16.716, 0.408) -> (16.716, -0.608)
  arc A1801 (16.6652, -0.608) -> (16.7668, -0.608) centre (16.716, -0.608) ccw
  arc A1802 (16.7668, 0.408) -> (16.6652, 0.408) centre (16.716, 0.408) ccw
  line L764 (16.716, -0.608) -> (14.684, -0.608)
  arc A1803 (14.684, -0.5572) -> (14.684, -0.6588) centre (14.684, -0.608) ccw
  arc A1804 (16.716, -0.6588) -> (16.716, -0.5572) centre (16.716, -0.608) ccw
  line L765 (14.684, -0.608) -> (14.684, 0.408)
  arc A1805 (14.7348, 0.408) -> (14.6332, 0.408) centre (14.684, 0.408) ccw
  arc A1806 (14.6332, -0.608) -> (14.7348, -0.608) centre (14.684, -0.608) ccw
  arc A1807 (66.8348, 40.108) -> (66.7332, 40.108) centre (66.784, 40.108) ccw
  line L766 (16.916, -4.608) -> (14.884, -4.608)
  arc A1808 (14.884, -4.5572) -> (14.884, -4.6588) centre (14.884, -4.608) ccw
  arc A1809 (16.916, -4.6588) -> (16.916, -4.5572) centre (16.916, -4.608) ccw
  line L767 (14.884, -4.608) -> (14.884, -3.592)
  arc A1810 (14.9348, -3.592) -> (14.8332, -3.592) centre (14.884, -3.592) ccw
  arc A1811 (14.8332, -4.608) -> (14.9348, -4.608) centre (14.884, -4.608) ccw
  line L768 (14.884, -3.592) -> (16.916, -3.592)
  arc A1812 (16.916, -3.6428) -> (16.916, -3.5412) centre (16.916, -3.592) ccw
  arc A1813 (14.884, -3.5412) -> (14.884, -3.6428) centre (14.884, -3.592) ccw
  line L769 (16.916, -3.592) -> (16.916, -4.608)
  arc A1814 (16.8652, -4.608) -> (16.9668, -4.608) centre (16.916, -4.608) ccw
  arc A1815 (16.9668, -3.592) -> (16.8652, -3.592) centre (16.916, -3.592) ccw
  arc A1816 (66.7332, 39.092) -> (66.8348, 39.092) centre (66.784, 39.092) ccw
  line L770 (22.884, -7.592) -> (24.916, -7.592)
  arc A1817 (24.916, -7.6428) -> (24.916, -7.5412) centre (24.916, -7.592) ccw
  arc A1818 (22.884, -7.5412) -> (22.884, -7.6428) centre (22.884, -7.592) ccw
  line L771 (24.916, -7.592) -> (24.916, -8.608)
  arc A1819 (24.8652, -8.608) -> (24.9668, -8.608) centre (24.916, -8.608) ccw
  arc A1820 (24.9668, -7.592) -> (24.8652, -7.592) centre (24.916, -7.592) ccw
  line L772 (24.916, -8.608) -> (22.884, -8.608)
  arc A1821 (22.884, -8.5572) -> (22.884, -8.6588) centre (22.884, -8.608) ccw
  arc A1822 (24.916, -8.6588) -> (24.916, -8.5572) centre (24.916, -8.608) ccw
  line L773 (22.884, -8.608) -> (22.884, -7.592)
  arc A1823 (22.9348, -7.592) -> (22.8332, -7.592) centre (22.884, -7.592) ccw
  arc A1824 (22.8332, -8.608) -> (22.9348, -8.608) centre (22.884, -8.608) ccw
  line L774 (66.784, 40.108) -> (68.816, 40.108)
  line L775 (14.684, -9.992) -> (16.716, -9.992)
  arc A1825 (16.716, -10.0428) -> (16.716, -9.9412) centre (16.716, -9.992) ccw
  arc A1826 (14.684, -9.9412) -> (14.684, -10.0428) centre (14.684, -9.992) ccw
  line L776 (16.716, -9.992) -> (16.716, -11.008)
  arc A1827 (16.6652, -11.008) -> (16.7668, -11.008) centre (16.716, -11.008) ccw
  arc A1828 (16.7668, -9.992) -> (16.6652, -9.992) centre (16.716, -9.992) ccw
  line L777 (16.716, -11.008) -> (14.684, -11.008)
  arc A1829 (14.684, -10.9572) -> (14.684, -11.0588) centre (14.684, -11.008) ccw
  arc A1830 (16.716, -11.0588) -> (16.716, -10.9572) centre (16.716, -11.008) ccw
  line L778 (14.684, -11.008) -> (14.684, -9.992)
  arc A1831 (14.7348, -9.992) -> (14.6332, -9.992) centre (14.684, -9.992) ccw
  arc A1832 (14.6332, -11.008) -> (14.7348, -11.008) centre (14.684, -11.008) ccw
  arc A1833 (68.816, 40.0572) -> (68.816, 40.1588) centre (68.816, 40.108) ccw
  line L779 (16.716, -15.008) -> (14.684, -15.008)
  arc A1834 (14.684, -14.9572) -> (14.684, -15.0588) centre (14.684, -15.008) ccw
  arc A1835 (16.716, -15.0588) -> (16.716, -14.9572) centre (16.716, -15.008) ccw
  line L780 (14.684, -15.008) -> (14.684, -13.992)
  arc A1836 (14.7348, -13.992) -> (14.6332, -13.992) centre (14.684, -13.992) ccw
  arc A1837 (14.6332, -15.008) -> (14.7348, -15.008) centre (14.684, -15.008) ccw
  line L781 (14.684, -13.992) -> (16.716, -13.992)
  arc A1838 (16.716, -14.0428) -> (16.716, -13.9412) centre (16.716, -13.992) ccw
  arc A1839 (14.684, -13.9412) -> (14.684, -14.0428) centre (14.684, -13.992) ccw
  line L782 (16.716, -13.992) -> (16.716, -15.008)
  arc A1840 (16.6652, -15.008) -> (16.7668, -15.008) centre (16.716, -15.008) ccw
  arc A1841 (16.7668, -13.992) -> (16.6652, -13.992) centre (16.716, -13.992) ccw
  arc A1842 (66.784, 40.1588) -> (66.784, 40.0572) centre (66.784, 40.108) ccw
  line L783 (22.884, -17.992) -> (24.916, -17.992)
  arc A1843 (24.916, -18.0428) -> (24.916, -17.9412) centre (24.916, -17.992) ccw
  arc A1844 (22.884, -17.9412) -> (22.884, -18.0428) centre (22.884, -17.992) ccw
  line L784 (24.916, -17.992) -> (24.916, -19.008)
  arc A1845 (24.8652, -19.008) -> (24.9668, -19.008) centre (24.916, -19.008) ccw
  arc A1846 (24.9668, -17.992) -> (24.8652, -17.992) centre (24.916, -17.992) ccw
  line L785 (24.916, -19.008) -> (22.884, -19.008)
  arc A1847 (22.884, -18.9572) -> (22.884, -19.0588) centre (22.884, -19.008) ccw
  arc A1848 (24.916, -19.0588) -> (24.916, -18.9572) centre (24.916, -19.008) ccw
  line L786 (22.884, -19.008) -> (22.884, -17.992)
  arc A1849 (22.9348, -17.992) -> (22.8332, -17.992) centre (22.884, -17.992) ccw
  arc A1850 (22.8332, -19.008) -> (22.9348, -19.008) centre (22.884, -19.008) ccw
  line L787 (68.816, 40.108) -> (68.816, 39.092)
  line L788 (18.884, -7.592) -> (20.916, -7.592)
  arc A1851 (20.916, -7.6428) -> (20.916, -7.5412) centre (20.916, -7.592) ccw
  arc A1852 (18.884, -7.5412) -> (18.884, -7.6428) centre (18.884, -7.592) ccw
  line L789 (20.916, -7.592) -> (20.916, -8.608)
  arc A1853 (20.8652, -8.608) -> (20.9668, -8.608) centre (20.916, -8.608) ccw
  arc A1854 (20.9668, -7.592) -> (20.8652, -7.592) centre (20.916, -7.592) ccw
  line L790 (20.916, -8.608) -> (18.884, -8.608)
  arc A1855 (18.884, -8.5572) -> (18.884, -8.6588) centre (18.884, -8.608) ccw
  arc A1856 (20.916, -8.6588) -> (20.916, -8.5572) centre (20.916, -8.608) ccw
  line L791 (18.884, -8.608) -> (18.884, -7.592)
  arc A1857 (18.9348, -7.592) -> (18.8332, -7.592) centre (18.884, -7.592) ccw
  arc A1858 (18.8332, -8.608) -> (18.9348, -8.608) centre (18.884, -8.608) ccw
  arc A1859 (68.7652, 39.092) -> (68.8668, 39.092) centre (68.816, 39.092) ccw
  line L792 (12.684, -3.592) -> (14.716, -3.592)
  arc A1860 (14.716, -3.6428) -> (14.716, -3.5412) centre (14.716, -3.592) ccw
  arc A1861 (12.684, -3.5412) -> (12.684, -3.6428) centre (12.684, -3.592) ccw
  line L793 (14.716, -3.592) -> (14.716, -4.608)
  arc A1862 (14.6652, -4.608) -> (14.7668, -4.608) centre (14.716, -4.608) ccw
  arc A1863 (14.7668, -3.592) -> (14.6652, -3.592) centre (14.716, -3.592) ccw
  line L794 (14.716, -4.608) -> (12.684, -4.608)
  arc A1864 (12.684, -4.5572) -> (12.684, -4.6588) centre (12.684, -4.608) ccw
  arc A1865 (14.716, -4.6588) -> (14.716, -4.5572) centre (14.716, -4.608) ccw
  line L795 (12.684, -4.608) -> (12.684, -3.592)
  arc A1866 (12.7348, -3.592) -> (12.6332, -3.592) centre (12.684, -3.592) ccw
  arc A1867 (12.6332, -4.608) -> (12.7348, -4.608) centre (12.684, -4.608) ccw
  arc A1868 (68.8668, 40.108) -> (68.7652, 40.108) centre (68.816, 40.108) ccw
  line L796 (20.884, 0.408) -> (22.916, 0.408)
  arc A1869 (22.916, 0.3572) -> (22.916, 0.4588) centre (22.916, 0.408) ccw
  arc A1870 (20.884, 0.4588) -> (20.884, 0.3572) centre (20.884, 0.408) ccw
  line L797 (22.916, 0.408) -> (22.916, -0.608)
  arc A1871 (22.8652, -0.608) -> (22.9668, -0.608) centre (22.916, -0.608) ccw
  arc A1872 (22.9668, 0.408) -> (22.8652, 0.408) centre (22.916, 0.408) ccw
  line L798 (22.916, -0.608) -> (20.884, -0.608)
  arc A1873 (20.884, -0.5572) -> (20.884, -0.6588) centre (20.884, -0.608) ccw
  arc A1874 (22.916, -0.6588) -> (22.916, -0.5572) centre (22.916, -0.608) ccw
  line L799 (20.884, -0.608) -> (20.884, 0.408)
  arc A1875 (20.9348, 0.408) -> (20.8332, 0.408) centre (20.884, 0.408) ccw
  arc A1876 (20.8332, -0.608) -> (20.9348, -0.608) centre (20.884, -0.608) ccw
  line L800 (66.784, 39.108) -> (68.816, 39.108)
  line L801 (18.884, -17.992) -> (20.916, -17.992)
  arc A1877 (20.916, -18.0428) -> (20.916, -17.9412) centre (20.916, -17.992) ccw
  arc A1878 (18.884, -17.9412) -> (18.884, -18.0428) centre (18.884, -17.992) ccw
  line L802 (20.916, -17.992) -> (20.916, -19.008)
  arc A1879 (20.8652, -19.008) -> (20.9668, -19.008) centre (20.916, -19.008) ccw
  arc A1880 (20.9668, -17.992) -> (20.8652, -17.992) centre (20.916, -17.992) ccw
  line L803 (20.916, -19.008) -> (18.884, -19.008)
  arc A1881 (18.884, -18.9572) -> (18.884, -19.0588) centre (18.884, -19.008) ccw
  arc A1882 (20.916, -19.0588) -> (20.916, -18.9572) centre (20.916, -19.008) ccw
  line L804 (18.884, -19.008) -> (18.884, -17.992)
  arc A1883 (18.9348, -17.992) -> (18.8332, -17.992) centre (18.884, -17.992) ccw
  arc A1884 (18.8332, -19.008) -> (18.9348, -19.008) centre (18.884, -19.008) ccw
  arc A1885 (68.816, 39.0572) -> (68.816, 39.1588) centre (68.816, 39.108) ccw
  line L805 (12.684, -13.992) -> (14.716, -13.992)
  arc A1886 (14.716, -14.0428) -> (14.716, -13.9412) centre (14.716, -13.992) ccw
  arc A1887 (12.684, -13.9412) -> (12.684, -14.0428) centre (12.684, -13.992) ccw
  line L806 (14.716, -13.992) -> (14.716, -15.008)
  arc A1888 (14.6652, -15.008) -> (14.7668, -15.008) centre (14.716, -15.008) ccw
  arc A1889 (14.7668, -13.992) -> (14.6652, -13.992) centre (14.716, -13.992) ccw
  line L807 (14.716, -15.008) -> (12.684, -15.008)
  arc A1890 (12.684, -14.9572) -> (12.684, -15.0588) centre (12.684, -15.008) ccw
  arc A1891 (14.716, -15.0588) -> (14.716, -14.9572) centre (14.716, -15.008) ccw
  line L808 (12.684, -15.008) -> (12.684, -13.992)
  arc A1892 (12.7348, -13.992) -> (12.6332, -13.992) centre (12.684, -13.992) ccw
  arc A1893 (12.6332, -15.008) -> (12.7348, -15.008) centre (12.684, -15.008) ccw
  arc A1894 (66.784, 39.1588) -> (66.784, 39.0572) centre (66.784, 39.108) ccw
  line L809 (20.884, -9.992) -> (22.916, -9.992)
  arc A1895 (22.916, -10.0428) -> (22.916, -9.9412) centre (22.916, -9.992) ccw
  arc A1896 (20.884, -9.9412) -> (20.884, -10.0428) centre (20.884, -9.992) ccw
  line L810 (22.916, -9.992) -> (22.916, -11.008)
  arc A1897 (22.8652, -11.008) -> (22.9668, -11.008) centre (22.916, -11.008) ccw
  arc A1898 (22.9668, -9.992) -> (22.8652, -9.992) centre (22.916, -9.992) ccw
  line L811 (22.916, -11.008) -> (20.884, -11.008)
  arc A1899 (20.884, -10.9572) -> (20.884, -11.0588) centre (20.884, -11.008) ccw
  arc A1900 (22.916, -11.0588) -> (22.916, -10.9572) centre (22.916, -11.008) ccw
  line L812 (20.884, -11.008) -> (20.884, -9.992)
  arc A1901 (20.9348, -9.992) -> (20.8332, -9.992) centre (20.884, -9.992) ccw
  arc A1902 (20.8332, -11.008) -> (20.9348, -11.008) centre (20.884, -11.008) ccw
  line L813 (68.816, 39.108) -> (68.816, 38.092)
  line L814 (22.884, 0.408) -> (24.916, 0.408)
  arc A1903 (24.916, 0.3572) -> (24.916, 0.4588) centre (24.916, 0.408) ccw
  arc A1904 (22.884, 0.4588) -> (22.884, 0.3572) centre (22.884, 0.408) ccw
  line L815 (24.916, 0.408) -> (24.916, -0.608)
  arc A1905 (24.8652, -0.608) -> (24.9668, -0.608) centre (24.916, -0.608) ccw
  arc A1906 (24.9668, 0.408) -> (24.8652, 0.408) centre (24.916, 0.408) ccw
  line L816 (24.916, -0.608) -> (22.884, -0.608)
  arc A1907 (22.884, -0.5572) -> (22.884, -0.6588) centre (22.884, -0.608) ccw
  arc A1908 (24.916, -0.6588) -> (24.916, -0.5572) centre (24.916, -0.608) ccw
  line L817 (22.884, -0.608) -> (22.884, 0.408)
  arc A1909 (22.9348, 0.408) -> (22.8332, 0.408) centre (22.884, 0.408) ccw
  arc A1910 (22.8332, -0.608) -> (22.9348, -0.608) centre (22.884, -0.608) ccw
  arc A1911 (68.7652, 38.092) -> (68.8668, 38.092) centre (68.816, 38.092) ccw
  line L818 (18.884, -3.592) -> (20.916, -3.592)
  arc A1912 (20.916, -3.6428) -> (20.916, -3.5412) centre (20.916, -3.592) ccw
  arc A1913 (18.884, -3.5412) -> (18.884, -3.6428) centre (18.884, -3.592) ccw
  line L819 (20.916, -3.592) -> (20.916, -4.608)
  arc A1914 (20.8652, -4.608) -> (20.9668, -4.608) centre (20.916, -4.608) ccw
  arc A1915 (20.9668, -3.592) -> (20.8652, -3.592) centre (20.916, -3.592) ccw
  line L820 (20.916, -4.608) -> (18.884, -4.608)
  arc A1916 (18.884, -4.5572) -> (18.884, -4.6588) centre (18.884, -4.608) ccw
  arc A1917 (20.916, -4.6588) -> (20.916, -4.5572) centre (20.916, -4.608) ccw
  line L821 (18.884, -4.608) -> (18.884, -3.592)
  arc A1918 (18.9348, -3.592) -> (18.8332, -3.592) centre (18.884, -3.592) ccw
  arc A1919 (18.8332, -4.608) -> (18.9348, -4.608) centre (18.884, -4.608) ccw
  arc A1920 (68.8668, 39.108) -> (68.7652, 39.108) centre (68.816, 39.108) ccw
  line L822 (16.684, 22.208) -> (18.716, 22.208)
  arc A1921 (18.716, 22.1572) -> (18.716, 22.2588) centre (18.716, 22.208) ccw
  arc A1922 (16.684, 22.2588) -> (16.684, 22.1572) centre (16.684, 22.208) ccw
  line L823 (18.716, 22.208) -> (18.716, 21.192)
  arc A1923 (18.6652, 21.192) -> (18.7668, 21.192) centre (18.716, 21.192) ccw
  arc A1924 (18.7668, 22.208) -> (18.6652, 22.208) centre (18.716, 22.208) ccw
  line L824 (18.716, 21.192) -> (16.684, 21.192)
  arc A1925 (16.684, 21.2428) -> (16.684, 21.1412) centre (16.684, 21.192) ccw
  arc A1926 (18.716, 21.1412) -> (18.716, 21.2428) centre (18.716, 21.192) ccw
  line L825 (16.684, 21.192) -> (16.684, 22.208)
  arc A1927 (16.7348, 22.208) -> (16.6332, 22.208) centre (16.684, 22.208) ccw
  arc A1928 (16.6332, 21.192) -> (16.7348, 21.192) centre (16.684, 21.192) ccw
  line L826 (68.816, 38.092) -> (66.784, 38.092)
  line L827 (18.716, 16.192) -> (16.684, 16.192)
  arc A1929 (16.684, 16.2428) -> (16.684, 16.1412) centre (16.684, 16.192) ccw
  arc A1930 (18.716, 16.1412) -> (18.716, 16.2428) centre (18.716, 16.192) ccw
  line L828 (16.684, 16.192) -> (16.684, 17.208)
  arc A1931 (16.7348, 17.208) -> (16.6332, 17.208) centre (16.684, 17.208) ccw
  arc A1932 (16.6332, 16.192) -> (16.7348, 16.192) centre (16.684, 16.192) ccw
  line L829 (16.684, 17.208) -> (18.716, 17.208)
  arc A1933 (18.716, 17.1572) -> (18.716, 17.2588) centre (18.716, 17.208) ccw
  arc A1934 (16.684, 17.2588) -> (16.684, 17.1572) centre (16.684, 17.208) ccw
  line L830 (18.716, 17.208) -> (18.716, 16.192)
  arc A1935 (18.6652, 16.192) -> (18.7668, 16.192) centre (18.716, 16.192) ccw
  arc A1936 (18.7668, 17.208) -> (18.6652, 17.208) centre (18.716, 17.208) ccw
  arc A1937 (66.784, 38.1428) -> (66.784, 38.0412) centre (66.784, 38.092) ccw
  line L831 (4.916, -23.808) -> (2.884, -23.808)
  arc A1938 (2.884, -23.7572) -> (2.884, -23.8588) centre (2.884, -23.808) ccw
  arc A1939 (4.916, -23.8588) -> (4.916, -23.7572) centre (4.916, -23.808) ccw
  line L832 (2.884, -23.808) -> (2.884, -22.792)
  arc A1940 (2.9348, -22.792) -> (2.8332, -22.792) centre (2.884, -22.792) ccw
  arc A1941 (2.8332, -23.808) -> (2.9348, -23.808) centre (2.884, -23.808) ccw
  line L833 (2.884, -22.792) -> (4.916, -22.792)
  arc A1942 (4.916, -22.8428) -> (4.916, -22.7412) centre (4.916, -22.792) ccw
  arc A1943 (2.884, -22.7412) -> (2.884, -22.8428) centre (2.884, -22.792) ccw
  line L834 (4.916, -22.792) -> (4.916, -23.808)
  arc A1944 (4.8652, -23.808) -> (4.9668, -23.808) centre (4.916, -23.808) ccw
  arc A1945 (4.9668, -22.792) -> (4.8652, -22.792) centre (4.916, -22.792) ccw
  arc A1946 (68.816, 38.0412) -> (68.816, 38.1428) centre (68.816, 38.092) ccw
  line L835 (7.116, -23.808) -> (5.084, -23.808)
  arc A1947 (5.084, -23.7572) -> (5.084, -23.8588) centre (5.084, -23.808) ccw
  arc A1948 (7.116, -23.8588) -> (7.116, -23.7572) centre (7.116, -23.808) ccw
  line L836 (5.084, -23.808) -> (5.084, -22.792)
  arc A1949 (5.1348, -22.792) -> (5.0332, -22.792) centre (5.084, -22.792) ccw
  arc A1950 (5.0332, -23.808) -> (5.1348, -23.808) centre (5.084, -23.808) ccw
  line L837 (5.084, -22.792) -> (7.116, -22.792)
  arc A1951 (7.116, -22.8428) -> (7.116, -22.7412) centre (7.116, -22.792) ccw
  arc A1952 (5.084, -22.7412) -> (5.084, -22.8428) centre (5.084, -22.792) ccw
  line L838 (7.116, -22.792) -> (7.116, -23.808)
  arc A1953 (7.0652, -23.808) -> (7.1668, -23.808) centre (7.116, -23.808) ccw
  arc A1954 (7.1668, -22.792) -> (7.0652, -22.792) centre (7.116, -22.792) ccw
  line L839 (66.784, 38.092) -> (66.784, 39.108)
  line L840 (-0.316, -18.792) -> (1.716, -18.792)
  arc A1955 (1.716, -18.8428) -> (1.716, -18.7412) centre (1.716, -18.792) ccw
  arc A1956 (-0.316, -18.7412) -> (-0.316, -18.8428) centre (-0.316, -18.792) ccw
  line L841 (1.716, -18.792) -> (1.716, -19.808)
  arc A1957 (1.6652, -19.808) -> (1.7668, -19.808) centre (1.716, -19.808) ccw
  arc A1958 (1.7668, -18.792) -> (1.6652, -18.792) centre (1.716, -18.792) ccw
  line L842 (1.716, -19.808) -> (-0.316, -19.808)
  arc A1959 (-0.316, -19.7572) -> (-0.316, -19.8588) centre (-0.316, -19.808) ccw
  arc A1960 (1.716, -19.8588) -> (1.716, -19.7572) centre (1.716, -19.808) ccw
  line L843 (-0.316, -19.808) -> (-0.316, -18.792)
  arc A1961 (-0.2652, -18.792) -> (-0.3668, -18.792) centre (-0.316, -18.792) ccw
  arc A1962 (-0.3668, -19.808) -> (-0.2652, -19.808) centre (-0.316, -19.808) ccw
  arc A1963 (66.8348, 39.108) -> (66.7332, 39.108) centre (66.784, 39.108) ccw
  line L844 (11.116, -15.808) -> (9.084, -15.808)
  arc A1964 (9.084, -15.7572) -> (9.084, -15.8588) centre (9.084, -15.808) ccw
  arc A1965 (11.116, -15.8588) -> (11.116, -15.7572) centre (11.116, -15.808) ccw
  line L845 (9.084, -15.808) -> (9.084, -14.792)
  arc A1966 (9.1348, -14.792) -> (9.0332, -14.792) centre (9.084, -14.792) ccw
  arc A1967 (9.0332, -15.808) -> (9.1348, -15.808) centre (9.084, -15.808) ccw
  line L846 (9.084, -14.792) -> (11.116, -14.792)
  arc A1968 (11.116, -14.8428) -> (11.116, -14.7412) centre (11.116, -14.792) ccw
  arc A1969 (9.084, -14.7412) -> (9.084, -14.8428) centre (9.084, -14.792) ccw